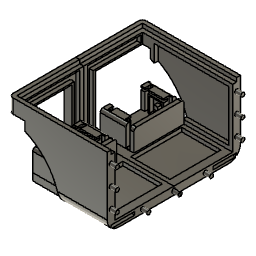
body ma v8 (Autodesk Fusion 360 design; units mm, degrees)
Autodesk Fusion 360 part; units mm, degrees
(part 1 of 2)
sketch "Sketch1" plane through (0, 0, 0) normal (0, 0, 1) x (1, 0, 0)
  line L0 (115, 75) -> (-115, 75)
  line L1 (-115, 75) -> (-115, -75)
  line L2 (-115, -75) -> (115, -75)
  line L3 (115, -75) -> (115, 75)
  line L4 (115, 75) -> (-115, -75) construction
  line L5 (-115, 75) -> (115, -75) construction
  line L6 (125, -85) -> (-125, -85)
  line L7 (-125, -85) -> (-125, 85)
  line L8 (-125, 85) -> (125, 85)
  line L9 (125, 85) -> (125, -85)
  line L10 (125, -85) -> (-125, 85) construction
  line L11 (-125, -85) -> (125, 85) construction
  line L12 (-125, 85) -> (-105, 85)
  line L13 (-105, 85) -> (-105, 20)
  line L14 (-110, 15) -> (-125, 15)
  line L15 (-125, 15) -> (-125, 85)
  line L16 (125, 85) -> (105, 85)
  line L17 (105, 85) -> (105, 20)
  line L18 (110, 15) -> (125, 15)
  line L19 (125, 15) -> (125, 85)
  line L20 (125, -85) -> (105, -85)
  line L21 (105, -85) -> (105, -20)
  line L22 (110, -15) -> (125, -15)
  line L23 (125, -15) -> (125, -85)
  line L24 (-125, -85) -> (-105, -85)
  line L25 (-105, -85) -> (-105, -20)
  line L26 (-110, -15) -> (-125, -15)
  line L27 (-125, -15) -> (-125, -85)
  arc A0 (-110, 15) -> (-105, 20) centre (-110, 20) ccw
  arc A1 (105, 20) -> (110, 15) centre (110, 20) ccw
  arc A2 (-105, -20) -> (-110, -15) centre (-110, -20) ccw
  arc A3 (110, -15) -> (105, -20) centre (110, -20) ccw
  dimension "d1" = 230
  dimension "d2" = 150
  dimension "d3" = 250
  dimension "d4" = 170
  dimension "d5" = 20
  dimension "d6" = 70
  dimension "d7" = 20
  dimension "d8" = 70
  dimension "d9" = 20
  dimension "d10" = 70
  dimension "d11" = 20
  dimension "d12" = 70
  dimension "d13" = 5
  dimension "d14" = 5
  dimension "d15" = 5
  dimension "d16" = 5
  constraint horizontal L0
  constraint perpendicular L0 L1
  constraint parallel L0 L2
  constraint parallel L1 L3
  constraint coincident L4 origin
  constraint coincident L5 origin
  constraint horizontal L6
  constraint perpendicular L6 L7
  constraint parallel L6 L8
  constraint parallel L7 L9
  constraint coincident L10 origin
  constraint coincident L11 origin
  constraint horizontal L12
  constraint vertical L13
  constraint horizontal L14
  constraint vertical L15
  constraint horizontal L16
  constraint vertical L17
  constraint horizontal L18
  constraint vertical L19
  constraint horizontal L20
  constraint vertical L21
  constraint horizontal L22
  constraint vertical L23
  constraint horizontal L24
  constraint vertical L25
  constraint horizontal L26
  constraint vertical L27
  constraint tangent L13 A0
  constraint tangent L14 A0
  constraint tangent L17 A1
  constraint tangent L18 A1
  constraint tangent L25 A2
  constraint tangent L26 A2
  constraint tangent L21 A3
  constraint tangent L22 A3
  measures "d1" distance of L1.end L2.end
  measures "d2" distance of L0.end L1.end
  measures "d3" distance of L7.end L8.end
  measures "d4" distance of L6.end L7.end
  measures "d5" distance of L7.end L12.end
  measures "d6" distance of L7.end L14.end
  measures "d7" distance of L8.end L16.end L10
  measures "d8" distance of L8.end L18.end L10
  measures "d9" distance of L6.start L20.end
  measures "d10" distance of L6.start L22.end
  measures "d11" distance of L6.end L24.end
  measures "d12" distance of L6.end L26.end
  measures "d13" radius of A0
  measures "d14" radius of A1
  measures "d15" radius of A2 L10
  measures "d16" radius of A3 L10
extrude "Extrude1" add sketch "Sketch1" along normal blind 10 contours L0 L1 L2 L3 L13 L14 L17 L18 L21 L22 L25 L26 A0 A1 A2 A3 | L0 L8 L13 L17 | L3 L9 L18 L22 | L1 L7 L14 L26 | L2 L6 L21 L25 makes body 1
extrude "Extrude2" add sketch "Sketch1" along normal blind 90 contours L0 L3 L8 L9 L16 L17 L18 L19 | L0 L8 L13 L17 | L3 L9 L18 L22 | L0 L1 L7 L8 L12 L13 L14 L15 | L2 L3 L6 L9 L20 L21 L22 L23 | L1 L7 L14 L26 | L2 L6 L21 L25 | L1 L2 L6 L7 L24 L25 L26 L27 bodies 1
extrude "Extrude3" cut sketch "Sketch1" along normal blind 72 contours L0 L3 L8 L9 L16 L17 L18 L19 | L0 L1 L7 L8 L12 L13 L14 L15 | L2 L3 L6 L9 L20 L21 L22 L23 | L1 L2 L6 L7 L24 L25 L26 L27 bodies 1
split "Split1" by plane through (0, 0, 0) normal (1, 0, 0) bodies 1 makes body 2 at (35.0675, 6.1971, 0)
sketch "Sketch2" plane through (0, 0, 0) normal (1, 0, 0) x (0, 1, 0)
  line L0 (75, 90) -> (75, 10)
  line L1 (75, 10) -> (-75, 10)
  line L2 (-75, 10) -> (-75, 90)
  line L3 (-75, 90) -> (-85, 90)
  line L4 (-85, 90) -> (-85, 0)
  line L5 (-85, 0) -> (85, 0)
  line L6 (85, 0) -> (85, 90)
  line L7 (85, 90) -> (75, 90)
  circle A0 centre (-80, 75) radius 2.5
  circle A1 centre (-80, 50) radius 2.5
  circle A2 centre (-80, 25) radius 2.5
  circle A3 centre (0, 5) radius 2.5
  circle A4 centre (-40, 5) radius 2.5
  circle A5 centre (40, 5) radius 2.5
  circle A6 centre (80, 25) radius 2.5
  circle A7 centre (80, 50) radius 2.5
  circle A8 centre (80, 75) radius 2.5
  dimension "d23" = 5
  dimension "d24" = 5
  dimension "d25" = 5
  dimension "d26" = 5
  dimension "d27" = 5
  dimension "d28" = 5
  dimension "d29" = 5
  dimension "d30" = 5
  dimension "d31" = 5
  dimension "d32" = 5
  dimension "d33" = 5
  dimension "d58" = 5
  dimension "d59" = 5
  dimension "d60" = 5
  dimension "d61" = 5
  dimension "d62" = 5
  dimension "d63" = 5
  dimension "d64" = 5
  dimension "d65" = 15
  dimension "d66" = 40
  dimension "d67" = 65
  dimension "d68" = 45
  dimension "d69" = 85
  dimension "d70" = 45
  dimension "d71" = 65
  dimension "d72" = 40
  dimension "d73" = 15
  measures "d23" diameter of A0
  measures "d24" diameter of A1
  measures "d25" diameter of A2
  measures "d26" diameter of A3
  measures "d27" diameter of A4
  measures "d28" diameter of A5
  measures "d29" diameter of A6
  measures "d30" diameter of A7
  measures "d31" diameter of A8
  measures "d32" distance of L4 A0.centre
  measures "d33" distance of L4 A1.centre
  measures "d58" distance of L4 A2.centre
  measures "d59" distance of L5 A4.centre
  measures "d60" distance of origin A3.centre
  measures "d61" distance of L5 A5.centre
  measures "d62" distance of L6 A6.centre
  measures "d63" distance of L6 A7.centre
  measures "d64" distance of L6 A8.centre
  measures "d65" distance of L3 A0.centre
  measures "d66" distance of L3 A1.centre
  measures "d67" distance of L3 A2.centre
  measures "d68" distance of L4 A4.centre
  measures "d69" distance of L4 A3.centre
  measures "d70" distance of L6 A5.centre
  measures "d71" distance of L7 A6.centre
  measures "d72" distance of L7 A7.centre
  measures "d73" distance of L7 A8.centre
extrude "Extrude4" add sketch "Sketch2" along normal blind 8 contours A0 | A1 | A2 | A3 | A4 | A5 | A6 | A7 | A8 bodies 1
sketch "Sketch3" plane through (0, 0, 0) normal (-1, 0, 0) x (0, -1, 0)
  line L0 (-75, 10) -> (-75, 90)
  line L1 (-75, 90) -> (-85, 90)
  line L2 (-85, 90) -> (-85, 0)
  line L3 (-85, 0) -> (85, 0)
  line L4 (85, 0) -> (85, 90)
  line L5 (85, 90) -> (75, 90)
  line L6 (75, 90) -> (75, 10)
  line L7 (75, 10) -> (-75, 10)
  circle A0 centre (-80, 75) radius 2.65
  circle A1 centre (-80, 50) radius 2.65
  circle A2 centre (-80, 25) radius 2.65
  circle A3 centre (-40, 5) radius 2.65
  circle A4 centre (0, 5) radius 2.65
  circle A5 centre (40, 5) radius 2.65
  circle A6 centre (80, 25) radius 2.65
  circle A7 centre (80, 50) radius 2.65
  circle A8 centre (80, 75) radius 2.65
  line L8 (50, 3) -> (80, 3)
  line L9 (80, 3) -> (80, 7)
  line L10 (80, 7) -> (50, 7)
  line L11 (50, 7) -> (50, 3)
  line L12 (50, 3) -> (80, 7) construction
  line L13 (80, 3) -> (50, 7) construction
  line L14 (-80, 3) -> (-50, 3)
  line L15 (-50, 3) -> (-50, 7)
  line L16 (-50, 7) -> (-80, 7)
  line L17 (-80, 7) -> (-80, 3)
  line L18 (-80, 3) -> (-50, 7) construction
  line L19 (-50, 3) -> (-80, 7) construction
  point P0 (65, 5)
  point P1 (-65, 5)
  dimension "d76" = 5.3
  dimension "d77" = 5.3
  dimension "d78" = 5.3
  dimension "d79" = 5.3
  dimension "d80" = 5.3
  dimension "d82" = 5.3
  dimension "d83" = 5.3
  dimension "d84" = 5.3
  dimension "d85" = 5.3
  dimension "d86" = 15
  dimension "d87" = 5
  dimension "d88" = 5
  dimension "d89" = 5
  dimension "d90" = 5
  dimension "d91" = 5
  dimension "d92" = 5
  dimension "d93" = 5
  dimension "d94" = 5
  dimension "d95" = 5
  dimension "d96" = 40
  dimension "d97" = 65
  dimension "d98" = 15
  dimension "d99" = 40
  dimension "d100" = 65
  dimension "d101" = 45
  dimension "d102" = 85
  dimension "d103" = 45
  dimension "d106" = 5
  dimension "d107" = 5
  dimension "d108" = 20
  dimension "d109" = 20
  dimension "d110" = 30
  dimension "d111" = 4
  dimension "d112" = 4
  dimension "d113" = 30
  constraint horizontal L8
  constraint perpendicular L8 L9
  constraint parallel L8 L10
  constraint parallel L9 L11
  constraint coincident L12 P0
  constraint coincident L13 P0
  constraint horizontal L14
  constraint perpendicular L14 L15
  constraint parallel L14 L16
  constraint parallel L15 L17
  constraint coincident L18 P1
  constraint coincident L19 P1
  measures "d76" diameter of A0
  measures "d77" diameter of A1
  measures "d78" diameter of A2
  measures "d79" diameter of A3
  measures "d80" diameter of A4
  measures "d82" diameter of A5
  measures "d83" diameter of A6
  measures "d84" diameter of A7
  measures "d85" diameter of A8
  measures "d86" distance of L1 A0.centre
  measures "d87" distance of L2 A0.centre
  measures "d88" distance of L2 A1.centre
  measures "d89" distance of L2 A2.centre
  measures "d90" distance of L3 A3.centre
  measures "d91" distance of L3 A4.centre
  measures "d92" distance of L3 A5.centre
  measures "d93" distance of L4 A6.centre
  measures "d94" distance of L4 A7.centre
  measures "d95" distance of L4 A8.centre
  measures "d96" distance of L1 A1.centre
  measures "d97" distance of L1 A2.centre
  measures "d98" distance of L5 A8.centre
  measures "d99" distance of L5 A7.centre
  measures "d100" distance of L5 A6.centre
  measures "d101" distance of L4 A5.centre
  measures "d102" distance of L4 A4.centre
  measures "d103" distance of L2 A3.centre
  measures "d106" distance of L7 P0
  measures "d107" distance of L7 P1
  measures "d108" distance of L2 P1
  measures "d109" distance of L4 P0
  measures "d110" distance of L9.end L10.end
  measures "d111" distance of L8.end L9.end
  measures "d112" distance of L14.start L16.end
  measures "d113" distance of L15.end L16.end
extrude "Extrude5" cut sketch "Sketch3" against normal blind 9 contours A0 | A1 | A2 | A3 | A4 | A5 | A6 | A7 | A8 bodies 2
extrude "Extrude6" cut sketch "Sketch3" along normal blind 8 contours L8 L9 L10 L11 | L14 L15 L16 L17 bodies 1
sketch "Sketch4" plane through (0, 0, 0) normal (-1, 0, 0) x (0, -1, 0)
  circle A0 centre (80, 25) radius 2.65
  circle A1 centre (-80, 25) radius 2.65
  circle A2 centre (-80, 50) radius 2.65
  circle A3 centre (40, 5) radius 2.65
  circle A4 centre (80, 50) radius 2.65
  circle A5 centre (-40, 5) radius 2.65
  circle A6 centre (-80, 75) radius 2.65
  circle A7 centre (0, 5) radius 2.65
  circle A8 centre (80, 75) radius 2.65
  line L0 (-75, 10) -> (-75, 90)
  line L1 (-75, 90) -> (-85, 90)
  line L2 (-85, 90) -> (-85, 0)
  line L3 (-85, 0) -> (85, 0)
  line L4 (85, 0) -> (85, 90)
  line L5 (85, 90) -> (75, 90)
  line L6 (75, 90) -> (75, 10)
  line L7 (75, 10) -> (-75, 10)
  line L8 (-51, 3.25) -> (-79, 3.25)
  line L9 (-79, 3.25) -> (-79, 6.75)
  line L10 (-79, 6.75) -> (-51, 6.75)
  line L11 (-51, 6.75) -> (-51, 3.25)
  line L12 (-51, 3.25) -> (-79, 6.75) construction
  line L13 (-79, 3.25) -> (-51, 6.75) construction
  line L14 (79, 3.25) -> (51, 3.25)
  line L15 (51, 3.25) -> (51, 6.75)
  line L16 (51, 6.75) -> (79, 6.75)
  line L17 (79, 6.75) -> (79, 3.25)
  line L18 (79, 3.25) -> (51, 6.75) construction
  line L19 (51, 3.25) -> (79, 6.75) construction
  point P0 (-65, 5)
  point P1 (65, 5)
  dimension "d116" = 20
  dimension "d117" = 5
  dimension "d118" = 5
  dimension "d119" = 20
  dimension "d120" = 28
  dimension "d121" = 3.5
  dimension "d122" = 28
  dimension "d123" = 3.5
  constraint horizontal L8
  constraint perpendicular L8 L9
  constraint parallel L8 L10
  constraint parallel L9 L11
  constraint coincident L12 P0
  constraint coincident L13 P0
  constraint horizontal L14
  constraint perpendicular L14 L15
  constraint parallel L14 L16
  constraint parallel L15 L17
  constraint coincident L18 P1
  constraint coincident L19 P1
  measures "d116" distance of L2 P0
  measures "d117" distance of L3 P0
  measures "d118" distance of L3 P1
  measures "d119" distance of L4 P1
  measures "d120" distance of L9.end L10.end
  measures "d121" distance of L8.end L9.end
  measures "d122" distance of L15.end L16.end
  measures "d123" distance of L14.start L16.end
extrude "Extrude7" add sketch "Sketch4" along normal blind 7.8 contours L8 L9 L10 L11 | L14 L15 L16 L17 bodies 2
fillet "Fillet1" radius 5 4 edges at (-125, 85, 81) (-125, -85, 81) (125, 85, 81) (125, -85, 81) on bodies 1 2
fillet "Fillet2" radius 15 2 edges at (-125, 0, 0) (125, 0, 0) on bodies 1 2
fillet "Fillet3" radius 15 4 edges at (-52.5, -85, 0) (-52.5, 85, 0) (52.5, -85, 0) (52.5, 85, 0) on bodies 1 2
sketch "Sketch5" plane through (0, 0, 90) normal (0, 0, 1) x (-1, 0, 0)
  arc A0 (125, 80) -> (120, 85) centre (120, 80) ccw
  line L0 (120, 85) -> (0, 85)
  line L1 (0, 85) -> (0, 75)
  line L2 (0, 75) -> (115, 75)
  line L3 (115, 75) -> (115, -75)
  line L4 (115, -75) -> (0, -75)
  line L5 (0, -75) -> (0, -85)
  line L6 (0, -85) -> (120, -85)
  arc A1 (120, -85) -> (125, -80) centre (120, -80) ccw
  line L7 (125, -80) -> (125, 80)
  line L8 (120, 80) -> (-120, 80)
  line L9 (-120, 80) -> (-120, -80)
  line L10 (-120, -80) -> (120, -80)
  line L11 (120, -80) -> (120, 80)
  line L12 (120, 80) -> (-120, -80) construction
  line L13 (-120, 80) -> (120, -80) construction
  dimension "d132" = 240
  dimension "d133" = 160
  constraint horizontal L8
  constraint perpendicular L8 L9
  constraint parallel L8 L10
  constraint parallel L9 L11
  constraint coincident L12 origin
  constraint coincident L13 origin
  measures "d132" distance of L9.end A1.centre
  measures "d133" distance of L8.end L9.end
extrude "Extrude8" cut sketch "Sketch5" against normal blind 5 contours L1 L2 L3 L4 L5 L8 L10 L11 | L1 L2 L3 L4 L5 L8 L9 L10 bodies 1 2
sketch "Sketch1 (2)" plane through (0, 0, 0) normal (0, 0, 1) x (1, 0, 0) in component "rest_casing v2"
  line L0 (-13.5, -7.7959) -> (9.5, -7.7959)
  line L1 (9.5, -7.7959) -> (9.5, -4.7959)
  line L2 (9.5, -4.7959) -> (19.5, -4.7959)
  line L3 (19.5, -4.7959) -> (19.5, 1.2041)
  line L4 (19.5, 1.2041) -> (26.5, 1.2041)
  line L5 (26.5, 1.2041) -> (26.5, 4.2041)
  line L6 (26.5, 4.2041) -> (19.5, 4.2041)
  line L7 (19.5, 4.2041) -> (19.5, 30.2041)
  line L8 (19.5, 30.2041) -> (-19.5, 30.2041)
  line L9 (-19.5, 30.2041) -> (-19.5, 4.2041)
  line L10 (-19.5, 4.2041) -> (-26.5, 4.2041)
  line L11 (-26.5, 4.2041) -> (-26.5, 1.2041)
  line L12 (-26.5, 1.2041) -> (-19.5, 1.2041)
  line L13 (-19.5, 1.2041) -> (-19.5, -4.7959)
  line L14 (-19.5, -4.7959) -> (-13.5, -4.7959)
  line L15 (-13.5, -4.7959) -> (-13.5, -7.7959)
  line L16 (-20, 0.7041) -> (-32, 0.7041)
  line L17 (-32, 0.7041) -> (-32, -4.2959)
  line L18 (-32, -4.2959) -> (-20, -4.2959)
  line L19 (-20, -4.2959) -> (-20, 0.7041)
  line L20 (-32, 0.7041) -> (-27, 0.7041)
  line L21 (-27, 0.7041) -> (-27, 38.7041)
  line L22 (-27, 38.7041) -> (-32, 38.7041)
  line L23 (-32, 38.7041) -> (-32, 0.7041)
  line L24 (-27, 38.7041) -> (27, 38.7041)
  line L25 (27, 38.7041) -> (27, 33.7041)
  line L26 (27, 33.7041) -> (-27, 33.7041)
  line L27 (-27, 33.7041) -> (-27, 38.7041)
  line L28 (20, 0.7041) -> (32, 0.7041)
  line L29 (32, 0.7041) -> (32, -4.2959)
  line L30 (32, -4.2959) -> (20, -4.2959)
  line L31 (20, -4.2959) -> (20, 0.7041)
  line L32 (32, 0.7041) -> (27, 0.7041)
  line L33 (27, 0.7041) -> (27, 38.7041)
  line L34 (27, 38.7041) -> (32, 38.7041)
  line L35 (32, 38.7041) -> (32, 0.7041)
  line L36 (27, 4.7041) -> (20, 4.7041)
  line L37 (20, 4.7041) -> (20, 22.7041)
  line L38 (20, 22.7041) -> (27, 22.7041)
  line L39 (27, 22.7041) -> (27, 4.7041)
  line L40 (-27, 4.7041) -> (-20, 4.7041)
  line L41 (-20, 4.7041) -> (-20, 24.7041)
  line L42 (-20, 24.7041) -> (-27, 24.7041)
  line L43 (-27, 24.7041) -> (-27, 4.7041)
  line L44 (-32, 38.7041) -> (32, 38.7041)
  line L45 (32, 38.7041) -> (32, -4.2959)
  line L46 (32, -4.2959) -> (-32, -4.2959)
  line L47 (-32, -4.2959) -> (-32, 38.7041)
  line L48 (-27, 33.7041) -> (-32, 33.7041)
  line L49 (-32, 33.7041) -> (-32, 28.7041)
  line L50 (-32, 28.7041) -> (-27, 28.7041)
  line L51 (-27, 28.7041) -> (-27, 33.7041)
  line L52 (27, 33.7041) -> (32, 33.7041)
  line L53 (32, 33.7041) -> (32, 28.7041)
  line L54 (32, 28.7041) -> (27, 28.7041)
  line L55 (27, 28.7041) -> (27, 33.7041)
  dimension "d34" = 0.5
  dimension "d35" = 0.5
  dimension "d36" = 5
  dimension "d37" = 12
  dimension "d38" = 0.5
  dimension "d39" = 3.5
  dimension "d40" = 5
  dimension "d41" = 0.5
  dimension "d42" = 0.5
  dimension "d43" = 12
  dimension "d44" = 5
  dimension "d45" = 0.5
  dimension "d46" = 0.5
  dimension "d47" = 0.5
  dimension "d48" = 18
  dimension "d49" = 0.5
  dimension "d50" = 0.5
  dimension "d51" = 20
  dimension "d56" = 5
  dimension "d57" = 5
  constraint horizontal L16
  constraint vertical L17
  constraint horizontal L18
  constraint vertical L19
  constraint horizontal L20
  constraint vertical L21
  constraint horizontal L22
  constraint vertical L23
  constraint horizontal L24
  constraint vertical L25
  constraint horizontal L26
  constraint vertical L27
  constraint horizontal L28
  constraint vertical L29
  constraint horizontal L30
  constraint vertical L31
  constraint horizontal L32
  constraint vertical L33
  constraint horizontal L34
  constraint vertical L35
  constraint horizontal L36
  constraint vertical L37
  constraint horizontal L38
  constraint vertical L39
  constraint coincident L33 L36.start
  constraint horizontal L40
  constraint vertical L41
  constraint horizontal L42
  constraint vertical L43
  constraint coincident L21 L40.start
  constraint horizontal L44
  constraint vertical L45
  constraint horizontal L46
  constraint vertical L47
  constraint horizontal L48
  constraint vertical L49
  constraint horizontal L50
  constraint vertical L51
  constraint coincident L47 L49.end
  constraint horizontal L52
  constraint vertical L53
  constraint horizontal L54
  constraint vertical L55
  constraint coincident L45 L53.end
  measures "d34" distance of L13 L19
  measures "d35" distance of L12 L16
  measures "d36" distance of L16.end L17.end
  measures "d37" distance of L17.end L18.end
  measures "d38" distance of L11 L21
  measures "d39" distance of L8 L26
  measures "d40" distance of L24.end L25.end
  measures "d41" distance of L4 L28
  measures "d42" distance of L3 L31
  measures "d43" distance of L29.end L30.end
  measures "d44" distance of L28.end L29.end
  measures "d45" distance of L5 L33
  measures "d46" distance of L6 L36
  measures "d47" distance of L7 L37
  measures "d48" distance of L36.end L37.end
  measures "d49" distance of L10 L40
  measures "d50" distance of L9 L41
  measures "d51" distance of L40 L42
  measures "d56" distance of L48 L50
  measures "d57" distance of L52 L54
extrude "Extrude1'" add sketch "Sketch1 (2)" against normal blind 1 separate body contours L3 L4 L5 L6 L7 L8 L9 L10 L11 L12 L13 L16 L19 L21 L26 L28 L31 L33 L36 L37 L38 L40 L41 L42 L46 L51 L55 | L3 L4 L5 L6 L7 L8 L9 L10 L11 L12 L13 L46 | L16 L17 L18 L19 L20 L46 L47 | L28 L29 L30 L31 L32 L45 L46 | L16 L20 L21 L23 L43 L47 L50 | L28 L32 L33 L35 L39 L45 L54 | L21 L23 L47 L48 L49 L50 L51 | L21 L40 L41 L42 L43 | L33 L35 L45 L52 L53 L54 L55 | L33 L36 L37 L38 L39 | L21 L22 L23 L27 L44 L47 L48 | L25 L33 L34 L35 L44 L45 L52 | L21 L24 L25 L26 L27 L33 L44 makes body 3 in component "rest_casing v2"
extrude "Extrude2'" add sketch "Sketch1 (2)" along normal blind 26 contours L16 L17 L18 L19 L20 L46 L47 | L28 L29 L30 L31 L32 L45 L46 | L16 L20 L21 L23 L43 L47 L50 | L28 L32 L33 L35 L39 L45 L54 | L21 L40 L41 L42 L43 | L33 L36 L37 L38 L39 | L21 L22 L23 L27 L44 L47 L48 | L25 L33 L34 L35 L44 L45 L52 | L21 L24 L25 L26 L27 L33 L44 bodies 3 in component "rest_casing v2"
sketch "Sketch2 (2)" plane through (0, -4.2959, 0) normal (0, -1, 0) x (1, 0, 0) in component "rest_casing v2"
  line L0 (20, 0) -> (-20, 0)
  line L1 (-20, 0) -> (-20, 26)
  line L2 (-20, 26) -> (-32, 26)
  line L3 (-32, 26) -> (-32, -1)
  line L4 (-32, -1) -> (32, -1)
  line L5 (32, -1) -> (32, 26)
  line L6 (32, 26) -> (20, 26)
  line L7 (20, 26) -> (20, 0)
  line L8 (-25, 24) -> (25, 24)
  line L9 (25, 24) -> (25, 21.5)
  line L10 (25, 21.5) -> (-25, 21.5)
  line L11 (-25, 21.5) -> (-25, 24)
  line L12 (-32, 26) -> (32, 26)
  dimension "d58_1" = 2.5
  dimension "d59_1" = 50
  dimension "d60_1" = 2
  dimension "d61_1" = 7
  constraint horizontal L8
  constraint vertical L9
  constraint horizontal L10
  constraint vertical L11
  measures "d58_1" distance of L8.start L10.end
  measures "d59_1" distance of L8.start L8.end
  measures "d60_1" distance of L8 L12
  measures "d61_1" distance of L5 L9
extrude "Extrude3'" cut sketch "Sketch2 (2)" against normal blind 40 contours L1 L7 L8 L10 | L7 L8 L9 L10 | L1 L8 L10 L11 bodies 3 in component "rest_casing v2"
sketch "Sketch1 (3)" plane through (0, -4.2959, 0) normal (0, -1, 0) x (1, 0, 0) in component "lid"
  line L0 (-20, 21.5) -> (-25, 21.5)
  line L1 (-25, 21.5) -> (-25, 24)
  line L2 (-25, 24) -> (-20, 24)
  line L3 (-20, 24) -> (-20, 26)
  line L4 (-20, 26) -> (-32, 26)
  line L5 (-32, 26) -> (-32, -1)
  line L6 (-32, -1) -> (32, -1)
  line L7 (32, -1) -> (32, 26)
  line L8 (32, 26) -> (20, 26)
  line L9 (20, 26) -> (20, 24)
  line L10 (20, 24) -> (25, 24)
  line L11 (25, 24) -> (25, 21.5)
  line L12 (25, 21.5) -> (20, 21.5)
  line L13 (20, 21.5) -> (20, 0)
  line L14 (20, 0) -> (-20, 0)
  line L15 (-20, 0) -> (-20, 21.5)
  line L16 (24.5, 21.75) -> (-24.5, 21.75)
  line L17 (-24.5, 21.75) -> (-24.5, 23.75)
  line L18 (-24.5, 23.75) -> (24.5, 23.75)
  line L19 (24.5, 23.75) -> (24.5, 21.75)
  line L20 (24.5, 21.75) -> (-24.5, 23.75) construction
  line L21 (-24.5, 21.75) -> (24.5, 23.75) construction
  point P0 (0, 22.75)
  dimension "d64_1" = 49
  dimension "d65_1" = 2
  dimension "d66_1" = 2.25
  dimension "d67_1" = 0.5
  constraint horizontal L16
  constraint perpendicular L16 L17
  constraint parallel L16 L18
  constraint parallel L17 L19
  constraint coincident L20 P0
  constraint coincident L21 P0
  measures "d64_1" distance of L17.end L18.end
  measures "d65_1" distance of L16.end L17.end
  measures "d66_1" distance of L8 L18
  measures "d67_1" distance of L11 L19
extrude "Extrude1''" add sketch "Sketch1 (3)" against normal blind 39 separate body contours L16 L17 L18 L19 makes body 4 in component "lid"
fillet "Fillet1'" radius 3.5 4 edges at (-32, 12.2041, 26) (32, 12.2041, 26) (32, 36.2041, 26) (-32, 36.2041, 26) on bodies 3 in component "rest_casing v2"
sketch "Sketch1 (4)" plane through (0, 0, 0) normal (0, 0, 1) x (1, 0, 0) in component "rest_casing v2 (1)"
  line L0 (-13.5, -7.7959) -> (9.5, -7.7959)
  line L1 (9.5, -7.7959) -> (9.5, -4.7959)
  line L2 (9.5, -4.7959) -> (19.5, -4.7959)
  line L3 (19.5, -4.7959) -> (19.5, 1.2041)
  line L4 (19.5, 1.2041) -> (26.5, 1.2041)
  line L5 (26.5, 1.2041) -> (26.5, 4.2041)
  line L6 (26.5, 4.2041) -> (19.5, 4.2041)
  line L7 (19.5, 4.2041) -> (19.5, 30.2041)
  line L8 (19.5, 30.2041) -> (-19.5, 30.2041)
  line L9 (-19.5, 30.2041) -> (-19.5, 4.2041)
  line L10 (-19.5, 4.2041) -> (-26.5, 4.2041)
  line L11 (-26.5, 4.2041) -> (-26.5, 1.2041)
  line L12 (-26.5, 1.2041) -> (-19.5, 1.2041)
  line L13 (-19.5, 1.2041) -> (-19.5, -4.7959)
  line L14 (-19.5, -4.7959) -> (-13.5, -4.7959)
  line L15 (-13.5, -4.7959) -> (-13.5, -7.7959)
  line L16 (-20, 0.7041) -> (-32, 0.7041)
  line L17 (-32, 0.7041) -> (-32, -4.2959)
  line L18 (-32, -4.2959) -> (-20, -4.2959)
  line L19 (-20, -4.2959) -> (-20, 0.7041)
  line L20 (-32, 0.7041) -> (-27, 0.7041)
  line L21 (-27, 0.7041) -> (-27, 38.7041)
  line L22 (-27, 38.7041) -> (-32, 38.7041)
  line L23 (-32, 38.7041) -> (-32, 0.7041)
  line L24 (-27, 38.7041) -> (27, 38.7041)
  line L25 (27, 38.7041) -> (27, 33.7041)
  line L26 (27, 33.7041) -> (-27, 33.7041)
  line L27 (-27, 33.7041) -> (-27, 38.7041)
  line L28 (20, 0.7041) -> (32, 0.7041)
  line L29 (32, 0.7041) -> (32, -4.2959)
  line L30 (32, -4.2959) -> (20, -4.2959)
  line L31 (20, -4.2959) -> (20, 0.7041)
  line L32 (32, 0.7041) -> (27, 0.7041)
  line L33 (27, 0.7041) -> (27, 38.7041)
  line L34 (27, 38.7041) -> (32, 38.7041)
  line L35 (32, 38.7041) -> (32, 0.7041)
  line L36 (27, 4.7041) -> (20, 4.7041)
  line L37 (20, 4.7041) -> (20, 22.7041)
  line L38 (20, 22.7041) -> (27, 22.7041)
  line L39 (27, 22.7041) -> (27, 4.7041)
  line L40 (-27, 4.7041) -> (-20, 4.7041)
  line L41 (-20, 4.7041) -> (-20, 24.7041)
  line L42 (-20, 24.7041) -> (-27, 24.7041)
  line L43 (-27, 24.7041) -> (-27, 4.7041)
  line L44 (-32, 38.7041) -> (32, 38.7041)
  line L45 (32, 38.7041) -> (32, -4.2959)
  line L46 (32, -4.2959) -> (-32, -4.2959)
  line L47 (-32, -4.2959) -> (-32, 38.7041)
  line L48 (-27, 33.7041) -> (-32, 33.7041)
  line L49 (-32, 33.7041) -> (-32, 28.7041)
  line L50 (-32, 28.7041) -> (-27, 28.7041)
  line L51 (-27, 28.7041) -> (-27, 33.7041)
  line L52 (27, 33.7041) -> (32, 33.7041)
  line L53 (32, 33.7041) -> (32, 28.7041)
  line L54 (32, 28.7041) -> (27, 28.7041)
  line L55 (27, 28.7041) -> (27, 33.7041)
  dimension "d34_1" = 0.5
  dimension "d35_1" = 0.5
  dimension "d36_1" = 5
  dimension "d37_1" = 12
  dimension "d38_1" = 0.5
  dimension "d39_1" = 3.5
  dimension "d40_1" = 5
  dimension "d41_1" = 0.5
  dimension "d42_1" = 0.5
  dimension "d43_1" = 12
  dimension "d44_1" = 5
  dimension "d45_1" = 0.5
  dimension "d46_1" = 0.5
  dimension "d47_1" = 0.5
  dimension "d48_1" = 18
  dimension "d49_1" = 0.5
  dimension "d50_1" = 0.5
  dimension "d51_1" = 20
  dimension "d56_1" = 5
  dimension "d57_1" = 5
  constraint horizontal L16
  constraint vertical L17
  constraint horizontal L18
  constraint vertical L19
  constraint horizontal L20
  constraint vertical L21
  constraint horizontal L22
  constraint vertical L23
  constraint horizontal L24
  constraint vertical L25
  constraint horizontal L26
  constraint vertical L27
  constraint horizontal L28
  constraint vertical L29
  constraint horizontal L30
  constraint vertical L31
  constraint horizontal L32
  constraint vertical L33
  constraint horizontal L34
  constraint vertical L35
  constraint horizontal L36
  constraint vertical L37
  constraint horizontal L38
  constraint vertical L39
  constraint coincident L33 L36.start
  constraint horizontal L40
  constraint vertical L41
  constraint horizontal L42
  constraint vertical L43
  constraint coincident L21 L40.start
  constraint horizontal L44
  constraint vertical L45
  constraint horizontal L46
  constraint vertical L47
  constraint horizontal L48
  constraint vertical L49
  constraint horizontal L50
  constraint vertical L51
  constraint coincident L47 L49.end
  constraint horizontal L52
  constraint vertical L53
  constraint horizontal L54
  constraint vertical L55
  constraint coincident L45 L53.end
  measures "d34_1" distance of L13 L19
  measures "d35_1" distance of L12 L16
  measures "d36_1" distance of L16.end L17.end
  measures "d37_1" distance of L17.end L18.end
  measures "d38_1" distance of L11 L21
  measures "d39_1" distance of L8 L26
  measures "d40_1" distance of L24.end L25.end
  measures "d41_1" distance of L4 L28
  measures "d42_1" distance of L3 L31
  measures "d43_1" distance of L29.end L30.end
  measures "d44_1" distance of L28.end L29.end
  measures "d45_1" distance of L5 L33
  measures "d46_1" distance of L6 L36
  measures "d47_1" distance of L7 L37
  measures "d48_1" distance of L36.end L37.end
  measures "d49_1" distance of L10 L40
  measures "d50_1" distance of L9 L41
  measures "d51_1" distance of L40 L42
  measures "d56_1" distance of L48 L50
  measures "d57_1" distance of L52 L54
extrude "Extrude1'''" add sketch "Sketch1 (4)" against normal blind 1 separate body contours L3 L4 L5 L6 L7 L8 L9 L10 L11 L12 L13 L16 L19 L21 L26 L28 L31 L33 L36 L37 L38 L40 L41 L42 L46 L51 L55 | L3 L4 L5 L6 L7 L8 L9 L10 L11 L12 L13 L46 | L16 L17 L18 L19 L20 L46 L47 | L28 L29 L30 L31 L32 L45 L46 | L16 L20 L21 L23 L43 L47 L50 | L28 L32 L33 L35 L39 L45 L54 | L21 L23 L47 L48 L49 L50 L51 | L21 L40 L41 L42 L43 | L33 L35 L45 L52 L53 L54 L55 | L33 L36 L37 L38 L39 | L21 L22 L23 L27 L44 L47 L48 | L25 L33 L34 L35 L44 L45 L52 | L21 L24 L25 L26 L27 L33 L44 makes body 5 in component "rest_casing v2 (1)"
extrude "Extrude2''" add sketch "Sketch1 (4)" along normal blind 26 contours L16 L17 L18 L19 L20 L46 L47 | L28 L29 L30 L31 L32 L45 L46 | L16 L20 L21 L23 L43 L47 L50 | L28 L32 L33 L35 L39 L45 L54 | L21 L40 L41 L42 L43 | L33 L36 L37 L38 L39 | L21 L22 L23 L27 L44 L47 L48 | L25 L33 L34 L35 L44 L45 L52 | L21 L24 L25 L26 L27 L33 L44 bodies 5 in component "rest_casing v2 (1)"
sketch "Sketch2 (3)" plane through (0, -4.2959, 0) normal (0, -1, 0) x (1, 0, 0) in component "rest_casing v2 (1)"
  line L0 (20, 0) -> (-20, 0)
  line L1 (-20, 0) -> (-20, 26)
  line L2 (-20, 26) -> (-32, 26)
  line L3 (-32, 26) -> (-32, -1)
  line L4 (-32, -1) -> (32, -1)
  line L5 (32, -1) -> (32, 26)
  line L6 (32, 26) -> (20, 26)
  line L7 (20, 26) -> (20, 0)
  line L8 (-25, 24) -> (25, 24)
  line L9 (25, 24) -> (25, 21.5)
  line L10 (25, 21.5) -> (-25, 21.5)
  line L11 (-25, 21.5) -> (-25, 24)
  line L12 (-32, 26) -> (32, 26)
  dimension "d58_2" = 2.5
  dimension "d59_2" = 50
  dimension "d60_2" = 2
  dimension "d61_2" = 7
  constraint horizontal L8
  constraint vertical L9
  constraint horizontal L10
  constraint vertical L11
  measures "d58_2" distance of L8.start L10.end
  measures "d59_2" distance of L8.start L8.end
  measures "d60_2" distance of L8 L12
  measures "d61_2" distance of L5 L9
extrude "Extrude3''" cut sketch "Sketch2 (3)" against normal blind 40 contours L1 L7 L8 L10 | L7 L8 L9 L10 | L1 L8 L10 L11 bodies 5 in component "rest_casing v2 (1)"
sketch "Sketch1 (5)" plane through (0, -4.2959, 0) normal (0, -1, 0) x (1, 0, 0) in component "lid (1)"
  line L0 (-20, 21.5) -> (-25, 21.5)
  line L1 (-25, 21.5) -> (-25, 24)
  line L2 (-25, 24) -> (-20, 24)
  line L3 (-20, 24) -> (-20, 26)
  line L4 (-20, 26) -> (-32, 26)
  line L5 (-32, 26) -> (-32, -1)
  line L6 (-32, -1) -> (32, -1)
  line L7 (32, -1) -> (32, 26)
  line L8 (32, 26) -> (20, 26)
  line L9 (20, 26) -> (20, 24)
  line L10 (20, 24) -> (25, 24)
  line L11 (25, 24) -> (25, 21.5)
  line L12 (25, 21.5) -> (20, 21.5)
  line L13 (20, 21.5) -> (20, 0)
  line L14 (20, 0) -> (-20, 0)
  line L15 (-20, 0) -> (-20, 21.5)
  line L16 (24.5, 21.75) -> (-24.5, 21.75)
  line L17 (-24.5, 21.75) -> (-24.5, 23.75)
  line L18 (-24.5, 23.75) -> (24.5, 23.75)
  line L19 (24.5, 23.75) -> (24.5, 21.75)
  line L20 (24.5, 21.75) -> (-24.5, 23.75) construction
  line L21 (-24.5, 21.75) -> (24.5, 23.75) construction
  point P0 (0, 22.75)
  dimension "d64_2" = 49
  dimension "d65_2" = 2
  dimension "d66_2" = 2.25
  dimension "d67_2" = 0.5
  constraint horizontal L16
  constraint perpendicular L16 L17
  constraint parallel L16 L18
  constraint parallel L17 L19
  constraint coincident L20 P0
  constraint coincident L21 P0
  measures "d64_2" distance of L17.end L18.end
  measures "d65_2" distance of L16.end L17.end
  measures "d66_2" distance of L8 L18
  measures "d67_2" distance of L11 L19
extrude "Extrude1''''" add sketch "Sketch1 (5)" against normal blind 39 separate body contours L16 L17 L18 L19 makes body 6 in component "lid (1)"
fillet "Fillet1''" radius 3.5 4 edges at (-32, 12.2041, 26) (32, 12.2041, 26) (32, 36.2041, 26) (-32, 36.2041, 26) on bodies 5 in component "rest_casing v2 (1)"
sketch "Sketch1 (6)" plane through (0, 0, 0) normal (0, 0, 1) x (1, 0, 0) in component "rest_casing v2 (2)"
  line L0 (-13.5, -7.7959) -> (9.5, -7.7959)
  line L1 (9.5, -7.7959) -> (9.5, -4.7959)
  line L2 (9.5, -4.7959) -> (19.5, -4.7959)
  line L3 (19.5, -4.7959) -> (19.5, 1.2041)
  line L4 (19.5, 1.2041) -> (26.5, 1.2041)
  line L5 (26.5, 1.2041) -> (26.5, 4.2041)
  line L6 (26.5, 4.2041) -> (19.5, 4.2041)
  line L7 (19.5, 4.2041) -> (19.5, 30.2041)
  line L8 (19.5, 30.2041) -> (-19.5, 30.2041)
  line L9 (-19.5, 30.2041) -> (-19.5, 4.2041)
  line L10 (-19.5, 4.2041) -> (-26.5, 4.2041)
  line L11 (-26.5, 4.2041) -> (-26.5, 1.2041)
  line L12 (-26.5, 1.2041) -> (-19.5, 1.2041)
  line L13 (-19.5, 1.2041) -> (-19.5, -4.7959)
  line L14 (-19.5, -4.7959) -> (-13.5, -4.7959)
  line L15 (-13.5, -4.7959) -> (-13.5, -7.7959)
  line L16 (-20, 0.7041) -> (-32, 0.7041)
  line L17 (-32, 0.7041) -> (-32, -4.2959)
  line L18 (-32, -4.2959) -> (-20, -4.2959)
  line L19 (-20, -4.2959) -> (-20, 0.7041)
  line L20 (-32, 0.7041) -> (-27, 0.7041)
  line L21 (-27, 0.7041) -> (-27, 38.7041)
  line L22 (-27, 38.7041) -> (-32, 38.7041)
  line L23 (-32, 38.7041) -> (-32, 0.7041)
  line L24 (-27, 38.7041) -> (27, 38.7041)
  line L25 (27, 38.7041) -> (27, 33.7041)
  line L26 (27, 33.7041) -> (-27, 33.7041)
  line L27 (-27, 33.7041) -> (-27, 38.7041)
  line L28 (20, 0.7041) -> (32, 0.7041)
  line L29 (32, 0.7041) -> (32, -4.2959)
  line L30 (32, -4.2959) -> (20, -4.2959)
  line L31 (20, -4.2959) -> (20, 0.7041)
  line L32 (32, 0.7041) -> (27, 0.7041)
  line L33 (27, 0.7041) -> (27, 38.7041)
  line L34 (27, 38.7041) -> (32, 38.7041)
  line L35 (32, 38.7041) -> (32, 0.7041)
  line L36 (27, 4.7041) -> (20, 4.7041)
  line L37 (20, 4.7041) -> (20, 22.7041)
  line L38 (20, 22.7041) -> (27, 22.7041)
  line L39 (27, 22.7041) -> (27, 4.7041)
  line L40 (-27, 4.7041) -> (-20, 4.7041)
  line L41 (-20, 4.7041) -> (-20, 24.7041)
  line L42 (-20, 24.7041) -> (-27, 24.7041)
  line L43 (-27, 24.7041) -> (-27, 4.7041)
  line L44 (-32, 38.7041) -> (32, 38.7041)
  line L45 (32, 38.7041) -> (32, -4.2959)
  line L46 (32, -4.2959) -> (-32, -4.2959)
  line L47 (-32, -4.2959) -> (-32, 38.7041)
  line L48 (-27, 33.7041) -> (-32, 33.7041)
  line L49 (-32, 33.7041) -> (-32, 28.7041)
  line L50 (-32, 28.7041) -> (-27, 28.7041)
  line L51 (-27, 28.7041) -> (-27, 33.7041)
  line L52 (27, 33.7041) -> (32, 33.7041)
  line L53 (32, 33.7041) -> (32, 28.7041)
  line L54 (32, 28.7041) -> (27, 28.7041)
  line L55 (27, 28.7041) -> (27, 33.7041)
  dimension "d34_2" = 0.5
  dimension "d35_2" = 0.5
  dimension "d36_2" = 5
  dimension "d37_2" = 12
  dimension "d38_2" = 0.5
  dimension "d39_2" = 3.5
  dimension "d40_2" = 5
  dimension "d41_2" = 0.5
  dimension "d42_2" = 0.5
  dimension "d43_2" = 12
  dimension "d44_2" = 5
  dimension "d45_2" = 0.5
  dimension "d46_2" = 0.5
  dimension "d47_2" = 0.5
  dimension "d48_2" = 18
  dimension "d49_2" = 0.5
  dimension "d50_2" = 0.5
  dimension "d51_2" = 20
  dimension "d56_2" = 5
  dimension "d57_2" = 5
  constraint horizontal L16
  constraint vertical L17
  constraint horizontal L18
  constraint vertical L19
  constraint horizontal L20
  constraint vertical L21
  constraint horizontal L22
  constraint vertical L23
  constraint horizontal L24
  constraint vertical L25
  constraint horizontal L26
  constraint vertical L27
  constraint horizontal L28
  constraint vertical L29
  constraint horizontal L30
  constraint vertical L31
  constraint horizontal L32
  constraint vertical L33
  constraint horizontal L34
  constraint vertical L35
  constraint horizontal L36
  constraint vertical L37
  constraint horizontal L38
  constraint vertical L39
  constraint coincident L33 L36.start
  constraint horizontal L40
  constraint vertical L41
  constraint horizontal L42
  constraint vertical L43
  constraint coincident L21 L40.start
  constraint horizontal L44
  constraint vertical L45
  constraint horizontal L46
  constraint vertical L47
  constraint horizontal L48
  constraint vertical L49
  constraint horizontal L50
  constraint vertical L51
  constraint coincident L47 L49.end
  constraint horizontal L52
  constraint vertical L53
  constraint horizontal L54
  constraint vertical L55
  constraint coincident L45 L53.end
  measures "d34_2" distance of L13 L19
  measures "d35_2" distance of L12 L16
  measures "d36_2" distance of L16.end L17.end
  measures "d37_2" distance of L17.end L18.end
  measures "d38_2" distance of L11 L21
  measures "d39_2" distance of L8 L26
  measures "d40_2" distance of L24.end L25.end
  measures "d41_2" distance of L4 L28
  measures "d42_2" distance of L3 L31
  measures "d43_2" distance of L29.end L30.end
  measures "d44_2" distance of L28.end L29.end
  measures "d45_2" distance of L5 L33
  measures "d46_2" distance of L6 L36
  measures "d47_2" distance of L7 L37
  measures "d48_2" distance of L36.end L37.end
  measures "d49_2" distance of L10 L40
  measures "d50_2" distance of L9 L41
  measures "d51_2" distance of L40 L42
  measures "d56_2" distance of L48 L50
  measures "d57_2" distance of L52 L54
extrude "Extrude1'''''" add sketch "Sketch1 (6)" against normal blind 1 separate body contours L3 L4 L5 L6 L7 L8 L9 L10 L11 L12 L13 L16 L19 L21 L26 L28 L31 L33 L36 L37 L38 L40 L41 L42 L46 L51 L55 | L3 L4 L5 L6 L7 L8 L9 L10 L11 L12 L13 L46 | L16 L17 L18 L19 L20 L46 L47 | L28 L29 L30 L31 L32 L45 L46 | L16 L20 L21 L23 L43 L47 L50 | L28 L32 L33 L35 L39 L45 L54 | L21 L23 L47 L48 L49 L50 L51 | L21 L40 L41 L42 L43 | L33 L35 L45 L52 L53 L54 L55 | L33 L36 L37 L38 L39 | L21 L22 L23 L27 L44 L47 L48 | L25 L33 L34 L35 L44 L45 L52 | L21 L24 L25 L26 L27 L33 L44 makes body 7 in component "rest_casing v2 (2)"
extrude "Extrude2'''" add sketch "Sketch1 (6)" along normal blind 26 contours L16 L17 L18 L19 L20 L46 L47 | L28 L29 L30 L31 L32 L45 L46 | L16 L20 L21 L23 L43 L47 L50 | L28 L32 L33 L35 L39 L45 L54 | L21 L40 L41 L42 L43 | L33 L36 L37 L38 L39 | L21 L22 L23 L27 L44 L47 L48 | L25 L33 L34 L35 L44 L45 L52 | L21 L24 L25 L26 L27 L33 L44 bodies 7 in component "rest_casing v2 (2)"
sketch "Sketch2 (4)" plane through (0, -4.2959, 0) normal (0, -1, 0) x (1, 0, 0) in component "rest_casing v2 (2)"
  line L0 (20, 0) -> (-20, 0)
  line L1 (-20, 0) -> (-20, 26)
  line L2 (-20, 26) -> (-32, 26)
  line L3 (-32, 26) -> (-32, -1)
  line L4 (-32, -1) -> (32, -1)
  line L5 (32, -1) -> (32, 26)
  line L6 (32, 26) -> (20, 26)
  line L7 (20, 26) -> (20, 0)
  line L8 (-25, 24) -> (25, 24)
  line L9 (25, 24) -> (25, 21.5)
  line L10 (25, 21.5) -> (-25, 21.5)
  line L11 (-25, 21.5) -> (-25, 24)
  line L12 (-32, 26) -> (32, 26)
  dimension "d58_3" = 2.5
  dimension "d59_3" = 50
  dimension "d60_3" = 2
  dimension "d61_3" = 7
  constraint horizontal L8
  constraint vertical L9
  constraint horizontal L10
  constraint vertical L11
  measures "d58_3" distance of L8.start L10.end
  measures "d59_3" distance of L8.start L8.end
  measures "d60_3" distance of L8 L12
  measures "d61_3" distance of L5 L9
extrude "Extrude3'''" cut sketch "Sketch2 (4)" against normal blind 40 contours L1 L7 L8 L10 | L7 L8 L9 L10 | L1 L8 L10 L11 bodies 7 in component "rest_casing v2 (2)"
sketch "Sketch1 (7)" plane through (0, -4.2959, 0) normal (0, -1, 0) x (1, 0, 0) in component "lid (2)"
  line L0 (-20, 21.5) -> (-25, 21.5)
  line L1 (-25, 21.5) -> (-25, 24)
  line L2 (-25, 24) -> (-20, 24)
  line L3 (-20, 24) -> (-20, 26)
  line L4 (-20, 26) -> (-32, 26)
  line L5 (-32, 26) -> (-32, -1)
  line L6 (-32, -1) -> (32, -1)
  line L7 (32, -1) -> (32, 26)
  line L8 (32, 26) -> (20, 26)
  line L9 (20, 26) -> (20, 24)
  line L10 (20, 24) -> (25, 24)
  line L11 (25, 24) -> (25, 21.5)
  line L12 (25, 21.5) -> (20, 21.5)
  line L13 (20, 21.5) -> (20, 0)
  line L14 (20, 0) -> (-20, 0)
  line L15 (-20, 0) -> (-20, 21.5)
  line L16 (24.5, 21.75) -> (-24.5, 21.75)
  line L17 (-24.5, 21.75) -> (-24.5, 23.75)
  line L18 (-24.5, 23.75) -> (24.5, 23.75)
  line L19 (24.5, 23.75) -> (24.5, 21.75)
  line L20 (24.5, 21.75) -> (-24.5, 23.75) construction
  line L21 (-24.5, 21.75) -> (24.5, 23.75) construction
  point P0 (0, 22.75)
  dimension "d64_3" = 49
  dimension "d65_3" = 2
  dimension "d66_3" = 2.25
  dimension "d67_3" = 0.5
  constraint horizontal L16
  constraint perpendicular L16 L17
  constraint parallel L16 L18
  constraint parallel L17 L19
  constraint coincident L20 P0
  constraint coincident L21 P0
  measures "d64_3" distance of L17.end L18.end
  measures "d65_3" distance of L16.end L17.end
  measures "d66_3" distance of L8 L18
  measures "d67_3" distance of L11 L19
extrude "Extrude1''''''" add sketch "Sketch1 (7)" against normal blind 39 separate body contours L16 L17 L18 L19 makes body 8 in component "lid (2)"
fillet "Fillet1'''" radius 3.5 4 edges at (-32, 12.2041, 26) (32, 12.2041, 26) (32, 36.2041, 26) (-32, 36.2041, 26) on bodies 7 in component "rest_casing v2 (2)"
sketch "Sketch1 (8)" plane through (0, 0, 0) normal (0, 0, 1) x (1, 0, 0) in component "rest_casing v2 (3)"
  line L0 (-13.5, -7.7959) -> (9.5, -7.7959)
  line L1 (9.5, -7.7959) -> (9.5, -4.7959)
  line L2 (9.5, -4.7959) -> (19.5, -4.7959)
  line L3 (19.5, -4.7959) -> (19.5, 1.2041)
  line L4 (19.5, 1.2041) -> (26.5, 1.2041)
  line L5 (26.5, 1.2041) -> (26.5, 4.2041)
  line L6 (26.5, 4.2041) -> (19.5, 4.2041)
  line L7 (19.5, 4.2041) -> (19.5, 30.2041)
  line L8 (19.5, 30.2041) -> (-19.5, 30.2041)
  line L9 (-19.5, 30.2041) -> (-19.5, 4.2041)
  line L10 (-19.5, 4.2041) -> (-26.5, 4.2041)
  line L11 (-26.5, 4.2041) -> (-26.5, 1.2041)
  line L12 (-26.5, 1.2041) -> (-19.5, 1.2041)
  line L13 (-19.5, 1.2041) -> (-19.5, -4.7959)
  line L14 (-19.5, -4.7959) -> (-13.5, -4.7959)
  line L15 (-13.5, -4.7959) -> (-13.5, -7.7959)
  line L16 (-20, 0.7041) -> (-32, 0.7041)
  line L17 (-32, 0.7041) -> (-32, -4.2959)
  line L18 (-32, -4.2959) -> (-20, -4.2959)
  line L19 (-20, -4.2959) -> (-20, 0.7041)
  line L20 (-32, 0.7041) -> (-27, 0.7041)
  line L21 (-27, 0.7041) -> (-27, 38.7041)
  line L22 (-27, 38.7041) -> (-32, 38.7041)
  line L23 (-32, 38.7041) -> (-32, 0.7041)
  line L24 (-27, 38.7041) -> (27, 38.7041)
  line L25 (27, 38.7041) -> (27, 33.7041)
  line L26 (27, 33.7041) -> (-27, 33.7041)
  line L27 (-27, 33.7041) -> (-27, 38.7041)
  line L28 (20, 0.7041) -> (32, 0.7041)
  line L29 (32, 0.7041) -> (32, -4.2959)
  line L30 (32, -4.2959) -> (20, -4.2959)
  line L31 (20, -4.2959) -> (20, 0.7041)
  line L32 (32, 0.7041) -> (27, 0.7041)
  line L33 (27, 0.7041) -> (27, 38.7041)
  line L34 (27, 38.7041) -> (32, 38.7041)
  line L35 (32, 38.7041) -> (32, 0.7041)
  line L36 (27, 4.7041) -> (20, 4.7041)
  line L37 (20, 4.7041) -> (20, 22.7041)
  line L38 (20, 22.7041) -> (27, 22.7041)
  line L39 (27, 22.7041) -> (27, 4.7041)
  line L40 (-27, 4.7041) -> (-20, 4.7041)
  line L41 (-20, 4.7041) -> (-20, 24.7041)
  line L42 (-20, 24.7041) -> (-27, 24.7041)
  line L43 (-27, 24.7041) -> (-27, 4.7041)
  line L44 (-32, 38.7041) -> (32, 38.7041)
  line L45 (32, 38.7041) -> (32, -4.2959)
  line L46 (32, -4.2959) -> (-32, -4.2959)
  line L47 (-32, -4.2959) -> (-32, 38.7041)
  line L48 (-27, 33.7041) -> (-32, 33.7041)
  line L49 (-32, 33.7041) -> (-32, 28.7041)
  line L50 (-32, 28.7041) -> (-27, 28.7041)
  line L51 (-27, 28.7041) -> (-27, 33.7041)
  line L52 (27, 33.7041) -> (32, 33.7041)
  line L53 (32, 33.7041) -> (32, 28.7041)
  line L54 (32, 28.7041) -> (27, 28.7041)
  line L55 (27, 28.7041) -> (27, 33.7041)
  dimension "d34_3" = 0.5
  dimension "d35_3" = 0.5
  dimension "d36_3" = 5
  dimension "d37_3" = 12
  dimension "d38_3" = 0.5
  dimension "d39_3" = 3.5
  dimension "d40_3" = 5
  dimension "d41_3" = 0.5
  dimension "d42_3" = 0.5
  dimension "d43_3" = 12
  dimension "d44_3" = 5
  dimension "d45_3" = 0.5
  dimension "d46_3" = 0.5
  dimension "d47_3" = 0.5
  dimension "d48_3" = 18
  dimension "d49_3" = 0.5
  dimension "d50_3" = 0.5
  dimension "d51_3" = 20
  dimension "d56_3" = 5
  dimension "d57_3" = 5
  constraint horizontal L16
  constraint vertical L17
  constraint horizontal L18
  constraint vertical L19
  constraint horizontal L20
  constraint vertical L21
  constraint horizontal L22
  constraint vertical L23
  constraint horizontal L24
  constraint vertical L25
  constraint horizontal L26
  constraint vertical L27
  constraint horizontal L28
  constraint vertical L29
  constraint horizontal L30
  constraint vertical L31
  constraint horizontal L32
  constraint vertical L33
  constraint horizontal L34
  constraint vertical L35
  constraint horizontal L36
  constraint vertical L37
  constraint horizontal L38
  constraint vertical L39
  constraint coincident L33 L36.start
  constraint horizontal L40
  constraint vertical L41
  constraint horizontal L42
  constraint vertical L43
  constraint coincident L21 L40.start
  constraint horizontal L44
  constraint vertical L45
  constraint horizontal L46
  constraint vertical L47
  constraint horizontal L48
  constraint vertical L49
  constraint horizontal L50
  constraint vertical L51
  constraint coincident L47 L49.end
  constraint horizontal L52
  constraint vertical L53
  constraint horizontal L54
  constraint vertical L55
  constraint coincident L45 L53.end
  measures "d34_3" distance of L13 L19
  measures "d35_3" distance of L12 L16
  measures "d36_3" distance of L16.end L17.end
  measures "d37_3" distance of L17.end L18.end
  measures "d38_3" distance of L11 L21
  measures "d39_3" distance of L8 L26
  measures "d40_3" distance of L24.end L25.end
  measures "d41_3" distance of L4 L28
  measures "d42_3" distance of L3 L31
  measures "d43_3" distance of L29.end L30.end
  measures "d44_3" distance of L28.end L29.end
  measures "d45_3" distance of L5 L33
  measures "d46_3" distance of L6 L36
  measures "d47_3" distance of L7 L37
  measures "d48_3" distance of L36.end L37.end
  measures "d49_3" distance of L10 L40
  measures "d50_3" distance of L9 L41
  measures "d51_3" distance of L40 L42
  measures "d56_3" distance of L48 L50
  measures "d57_3" distance of L52 L54
extrude "Extrude1'''''''" add sketch "Sketch1 (8)" against normal blind 1 separate body contours L3 L4 L5 L6 L7 L8 L9 L10 L11 L12 L13 L16 L19 L21 L26 L28 L31 L33 L36 L37 L38 L40 L41 L42 L46 L51 L55 | L3 L4 L5 L6 L7 L8 L9 L10 L11 L12 L13 L46 | L16 L17 L18 L19 L20 L46 L47 | L28 L29 L30 L31 L32 L45 L46 | L16 L20 L21 L23 L43 L47 L50 | L28 L32 L33 L35 L39 L45 L54 | L21 L23 L47 L48 L49 L50 L51 | L21 L40 L41 L42 L43 | L33 L35 L45 L52 L53 L54 L55 | L33 L36 L37 L38 L39 | L21 L22 L23 L27 L44 L47 L48 | L25 L33 L34 L35 L44 L45 L52 | L21 L24 L25 L26 L27 L33 L44 makes body 9 in component "rest_casing v2 (3)"
extrude "Extrude2''''" add sketch "Sketch1 (8)" along normal blind 26 contours L16 L17 L18 L19 L20 L46 L47 | L28 L29 L30 L31 L32 L45 L46 | L16 L20 L21 L23 L43 L47 L50 | L28 L32 L33 L35 L39 L45 L54 | L21 L40 L41 L42 L43 | L33 L36 L37 L38 L39 | L21 L22 L23 L27 L44 L47 L48 | L25 L33 L34 L35 L44 L45 L52 | L21 L24 L25 L26 L27 L33 L44 bodies 9 in component "rest_casing v2 (3)"
sketch "Sketch2 (5)" plane through (0, -4.2959, 0) normal (0, -1, 0) x (1, 0, 0) in component "rest_casing v2 (3)"
  line L0 (20, 0) -> (-20, 0)
  line L1 (-20, 0) -> (-20, 26)
  line L2 (-20, 26) -> (-32, 26)
  line L3 (-32, 26) -> (-32, -1)
  line L4 (-32, -1) -> (32, -1)
  line L5 (32, -1) -> (32, 26)
  line L6 (32, 26) -> (20, 26)
  line L7 (20, 26) -> (20, 0)
  line L8 (-25, 24) -> (25, 24)
  line L9 (25, 24) -> (25, 21.5)
  line L10 (25, 21.5) -> (-25, 21.5)
  line L11 (-25, 21.5) -> (-25, 24)
  line L12 (-32, 26) -> (32, 26)
  dimension "d58_4" = 2.5
  dimension "d59_4" = 50
  dimension "d60_4" = 2
  dimension "d61_4" = 7
  constraint horizontal L8
  constraint vertical L9
  constraint horizontal L10
  constraint vertical L11
  measures "d58_4" distance of L8.start L10.end
  measures "d59_4" distance of L8.start L8.end
  measures "d60_4" distance of L8 L12
  measures "d61_4" distance of L5 L9
extrude "Extrude3''''" cut sketch "Sketch2 (5)" against normal blind 40 contours L1 L7 L8 L10 | L7 L8 L9 L10 | L1 L8 L10 L11 bodies 9 in component "rest_casing v2 (3)"
sketch "Sketch1 (9)" plane through (0, -4.2959, 0) normal (0, -1, 0) x (1, 0, 0) in component "lid (3)"
  line L0 (-20, 21.5) -> (-25, 21.5)
  line L1 (-25, 21.5) -> (-25, 24)
  line L2 (-25, 24) -> (-20, 24)
  line L3 (-20, 24) -> (-20, 26)
  line L4 (-20, 26) -> (-32, 26)
  line L5 (-32, 26) -> (-32, -1)
  line L6 (-32, -1) -> (32, -1)
  line L7 (32, -1) -> (32, 26)
  line L8 (32, 26) -> (20, 26)
  line L9 (20, 26) -> (20, 24)
  line L10 (20, 24) -> (25, 24)
  line L11 (25, 24) -> (25, 21.5)
  line L12 (25, 21.5) -> (20, 21.5)
  line L13 (20, 21.5) -> (20, 0)
  line L14 (20, 0) -> (-20, 0)
  line L15 (-20, 0) -> (-20, 21.5)
  line L16 (24.5, 21.75) -> (-24.5, 21.75)
  line L17 (-24.5, 21.75) -> (-24.5, 23.75)
  line L18 (-24.5, 23.75) -> (24.5, 23.75)
  line L19 (24.5, 23.75) -> (24.5, 21.75)
  line L20 (24.5, 21.75) -> (-24.5, 23.75) construction
  line L21 (-24.5, 21.75) -> (24.5, 23.75) construction
  point P0 (0, 22.75)
  dimension "d64_4" = 49
  dimension "d65_4" = 2
  dimension "d66_4" = 2.25
  dimension "d67_4" = 0.5
  constraint horizontal L16
  constraint perpendicular L16 L17
  constraint parallel L16 L18
  constraint parallel L17 L19
  constraint coincident L20 P0
  constraint coincident L21 P0
  measures "d64_4" distance of L17.end L18.end
  measures "d65_4" distance of L16.end L17.end
  measures "d66_4" distance of L8 L18
  measures "d67_4" distance of L11 L19
extrude "Extrude1''''''''" add sketch "Sketch1 (9)" against normal blind 39 separate body contours L16 L17 L18 L19 makes body 10 in component "lid (3)"
fillet "Fillet1''''" radius 3.5 4 edges at (-32, 12.2041, 26) (32, 12.2041, 26) (32, 36.2041, 26) (-32, 36.2041, 26) on bodies 9 in component "rest_casing v2 (3)"
delete_body "RemoveBody1" bodies 2